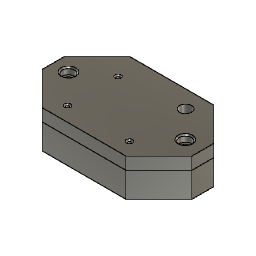
feet mold (Autodesk Fusion 360 design; units mm, degrees)
Autodesk Fusion 360 part; units mm, degrees
note: some values were not read from the file. Chosen so that the rebuilt part matches the saved one: which bodies a step acts on; which face or edge a step refers to. Set by a fixed rule: which sketch regions a step uses.
sketch "base" plane through (0, 0, 0) normal (0, 0, 1) x (1, 0, 0)
  circle A0 centre (0, 0) radius 2.65
  circle A1 centre (0, 0) radius 5
  line L0 (-10, 18.1) -> (18.1, 18.1)
  line L1 (18.1, 18.1) -> (18.1, -10)
  line L2 (18.1, -10) -> (-10, -10)
  line L3 (-10, -10) -> (-10, 18.1)
  line L4 (0, 0) -> (0, 20) construction
  arc A2 (-4.8405, 18.1) -> (4.8405, 18.1) centre (0, 20) ccw
  line L5 (-10, 15.5) -> (-7.4, 18.1)
  line L6 (-10, -7.4) -> (-7.4, -10)
  line L7 (18.1, -7.4) -> (15.5, -10)
  line L8 (-10, -7.4) -> (18.1, -7.4) construction
  line L9 (-7.4, 18.1) -> (-7.4, -10) construction
  arc A3 (18.1, 4.8405) -> (18.1, -4.8405) centre (20, 0) ccw
  line L10 (0, 0) -> (20, 0) construction
  line L11 (-2.2249, 15.3) -> (2.2249, 15.3)
  line L12 (15.3, 2.2249) -> (15.3, -2.2249)
  line L13 (-30, 26) -> (38.1, 26)
  line L14 (38.1, 26) -> (38.1, -14)
  line L15 (38.1, -14) -> (-30, -14)
  line L16 (-30, -14) -> (-30, 26)
  circle A4 centre (-23, 6) radius 2.75
  circle A5 centre (-23, 6) radius 1.6
  line L17 (-19.7, 6) -> (-21.35, 8.8579)
  line L18 (-21.35, 8.8579) -> (-24.65, 8.8579)
  line L19 (-24.65, 8.8579) -> (-26.3, 6)
  line L20 (-26.3, 6) -> (-24.65, 3.1421)
  line L21 (-24.65, 3.1421) -> (-21.35, 3.1421)
  line L22 (-21.35, 3.1421) -> (-19.7, 6)
  circle A6 centre (30.1, 6) radius 1.6
  circle A7 centre (30.1, 6) radius 2.75
  line L23 (33.4, 6) -> (31.75, 8.8579)
  line L24 (31.75, 8.8579) -> (28.45, 8.8579)
  line L25 (28.45, 8.8579) -> (26.8, 6)
  line L26 (26.8, 6) -> (28.45, 3.1421)
  line L27 (28.45, 3.1421) -> (31.75, 3.1421)
  line L28 (31.75, 3.1421) -> (33.4, 6)
  circle A8 centre (-10, 15.5) radius 0.75
  circle A9 centre (-10, -7.4) radius 0.75
  circle A10 centre (18.1, 18.1) radius 2.325
  circle A11 centre (18.1, -7.4) radius 0.75
  point P0 (-23, 6)
  point P1 (30.1, 6)
  dimension "d5" = 5.3
  dimension "d6" = 10
  dimension "d7" = 10
  dimension "d12" = 10
  dimension "d13" = 5.2
  dimension "d14" = 2.6
  dimension "d27" = 20
  dimension "d59" = 45
  dimension "d61" = 45
  dimension "d62" = 45
  dimension "d68" = 5.2
  dimension "d69" = 20
  dimension "d70" = 28.1
  dimension "d81" = 1.9
  dimension "d88" = 0.5
  dimension "d89" = 0.5
  dimension "d94" = 25.5
  dimension "d95" = 68.1
  dimension "d96" = 40
  dimension "d97" = 20
  dimension "d107" = 5.5
  dimension "d108" = 3.2
  dimension "d109" = 3.3
  dimension "d110" = 3.2
  dimension "d111" = 5.5
  dimension "d112" = 3.3
  dimension "d113" = 20
  dimension "d114" = 20
  dimension "d115" = 7
  dimension "d116" = 8
  dimension "d127" = 1.5
  dimension "d128" = 1.5
  dimension "d130" = 4.65
  dimension "d139" = 1.5
  constraint coincident A0.centre A1.centre
  constraint concentric A0 A1
  constraint horizontal L0
  constraint vertical L1
  constraint horizontal L2
  constraint vertical L3
  constraint perpendicular L0 L4
  constraint coincident L0 A2.end
  constraint coincident L0 A2.start
  constraint coincident L4.end A2.centre
  constraint coincident L3 L5.start
  constraint coincident L0 L5.end
  constraint coincident L2 L6.end
  constraint coincident L3 L6.start
  constraint coincident L2 L7.end
  constraint coincident L1 L7.start
  constraint perpendicular L3 L8
  constraint perpendicular L2 L9
  constraint coincident L1 A3.end
  constraint coincident L1 A3.start
  constraint coincident A3.centre L10.end
  constraint perpendicular L4 L10
  constraint equal L2 L3
  constraint coincident A2 L11.end
  constraint perpendicular L4 L11
  constraint coincident A2 L11.start
  constraint coincident A3 L12.start
  constraint coincident A3 L12.end
  constraint perpendicular L10 L12
  constraint horizontal L13
  constraint vertical L14
  constraint horizontal L15
  constraint vertical L16
  constraint concentric A4 A5
  constraint coincident P0 A4.centre
  constraint concentric A6 A7
  constraint coincident P1 A6.centre
  constraint coincident L5.start A8.centre
  constraint coincident L6.start L8.start
  constraint coincident L0.end L1.start
  constraint coincident L7.start L8.end
  measures "d5" diameter of A0
  measures "d6" diameter of A1
  measures "d7" vertical distance of A0.centre L1.end
  measures "d12" horizontal distance of L0.start L4.end
  measures "d13" radius of A2
  measures "d14" horizontal distance of L0.start L5.end
  measures "d27" vertical distance of A0.centre L4.end
  measures "d59" angle of L2 L7
  measures "d61" angle of L0 L5
  measures "d62" angle of L2 L6
  measures "d68" radius of A3
  measures "d69" distance of A0.centre A3.centre
  measures "d70" distance of L0.start L2.end
  measures "d81" distance of L0 L4.end
  measures "d88" distance of A2 L11
  measures "d89" distance of A3 L12
  measures "d94" distance of L0.start L6.start
  measures "d95" distance of L13.start L13.end
  measures "d96" distance of L13.start L15.end
  measures "d97" distance of L3 L16
  measures "d107" diameter of A4
  measures "d108" diameter of A5
  measures "d109" distance of L17.start P0
  measures "d110" diameter of A6
  measures "d111" diameter of A7
  measures "d112" distance of L23.start P1
  measures "d113" distance of L15 P1
  measures "d114" distance of L15 P0
  measures "d115" distance of L16 P0
  measures "d116" distance of L14 P1
  measures "d127" diameter of A8
  measures "d128" diameter of A9
  measures "d130" diameter of A10
  measures "d139" diameter of A11
extrude "Extrude1" add sketch "base" along normal blind 6.4 contours L0 L1 L2 L3 A2 L5 L6 L7 A3 A8 A9 A10 A11 | L3 L5 A8 | A2 L11 | L3 L6 A9 | L0 L1 A10 | A3 L12 | L1 L7 A11 picked at (-9.6473, 15.1473) picked at (-9.6007, -7.1011) picked at (16.5579, 17.9897) picked at (18.0633, -6.9027) makes body 1
extrude "Extrude2" add sketch "base" along normal blind 3 contours A1 bodies 1
extrude "Extrude3" add sketch "base" along normal blind 2.6 contours L0 L3 L5 A8 | L0 L1 L2 L3 A2 L5 L6 L7 A3 A8 A9 A10 A11 | L3 L5 A8 | L0 A2 L11 | L3 L5 A8 | A2 L11 | L3 L6 A9 | L0 L1 A10 | L3 L6 A9 | L2 L3 L6 A9 | L1 A3 L12 | A3 L12 | L1 L2 L7 A11 | L1 L7 A11 | L1 L7 A11 picked at (16.5579, 17.9897) bodies 1
extrude "Extrude11" cut sketch "base" along normal up to surface (5.4 mm away) contours L0 A2 L11 | A2 L11 | L1 A3 L12 | A3 L12 bodies 1
draft "Draft2" angle 45 neutral plane through (-10, -7.4, 0) pull (-0.707107, -0.707107, 0) 1 faces at (-9.1333, -9.1333, 2.6) on bodies 1
draft "Draft3" angle 45 neutral plane through (18.1, -7.4, 0) pull (0.707107, -0.707107, 0) 1 faces at (17.2333, -9.1333, 2.6) on bodies 1
draft "Draft5" angle 45 neutral plane through (-10, 15.5, 0) pull (-0.707107, 0.707107, 0) 1 faces at (-9.1333, 17.2333, 2.6) on bodies 1
draft "Draft8" angle 45 neutral plane through (15.3, 2.2249, 0) pull (1, 0, 0) 1 faces at (15.2081, 0.5035, 5.4) on bodies 1
draft "Draft9" angle 45 neutral plane through (-2.2249, 15.3, 0) pull (0, 1, 0) 1 faces at (0.5035, 15.2081, 5.4) on bodies 1
sketch "selective_infill" plane through (0, 0, 0) normal (0, 0, -1) x (1, 0, 0)
  line L0 (-10, -18.1) -> (-4.8405, -18.1)
  line L1 (18.1, 4.8405) -> (18.1, 10)
  line L2 (18.1, 10) -> (-10, 10)
  line L3 (-10, 10) -> (-10, -18.1)
  circle A0 centre (0, 0) radius 2.65
  line L4 (4.7284, 2.65) -> (4.8294, 2.65)
  line L5 (4.8294, 2.65) -> (4.8294, -2.65)
  line L6 (4.8294, -2.65) -> (4.7284, -2.65)
  line L7 (4.7284, -2.65) -> (4.7284, 2.65)
  line L8 (-4.7284, 2.65) -> (-4.8294, 2.65)
  line L9 (-4.8294, 2.65) -> (-4.8294, -2.65)
  line L10 (-4.8294, -2.65) -> (-4.7284, -2.65)
  line L11 (-4.7284, -2.65) -> (-4.7284, 2.65)
  line L12 (-4.7284, 0) -> (4.7284, 0) construction
  arc A1 (18.1, 4.8405) -> (18.1, -4.8405) centre (20, 0) ccw
  arc A2 (4.8405, -18.1) -> (-4.8405, -18.1) centre (0, -20) ccw
  circle A3 centre (0, 0) radius 2.65
  line L13 (4.8405, -18.1) -> (18.1, -18.1)
  line L14 (18.1, -18.1) -> (18.1, -4.8405)
  dimension "d52" = 0.101
  dimension "d53" = 0.101
  constraint horizontal L4
  constraint vertical L5
  constraint horizontal L6
  constraint vertical L7
  constraint horizontal L8
  constraint vertical L9
  constraint horizontal L10
  constraint vertical L11
  constraint midpoint L11 L12.start
  constraint midpoint L7 L12.end
  constraint perpendicular L7 L12
  constraint coincident A0.centre L12
  constraint tangent A0 L10
  constraint tangent A0 L6
  measures "d52" distance of L8.start L8.end
  measures "d53" horizontal distance of L4.start L4.end
extrude "Extrude9" cut sketch "selective_infill" along normal up to surface (0.8 mm away) from surface at -1.8 contours L4 L5 L6 L7 | L8 L9 L10 L11 bodies 1
extrude "Extrude12" add sketch "base" against normal blind 5 separate body contours A0 | A1 | L0 L3 L5 A8 | L0 L1 L2 L3 A2 L5 L6 L7 A3 A8 A9 A10 A11 | L3 L5 A8 | L3 A8 | L0 A2 L11 | L3 L5 A8 | A2 L11 | L3 L6 A9 | L3 A9 | L0 L1 A10 | L0 L1 A10 | L3 L6 A9 | L2 L3 L6 A9 | L1 A3 L12 | A3 L12 | L1 L2 L7 A11 | L1 A11 | L1 L7 A11 | L1 L7 A11 | L13 L14 L15 L16 | A4 | A5 | L17 L18 L19 L20 L21 L22 | A6 | A7 | L23 L24 L25 L26 L27 L28 makes body 2
extrude "Extrude13" add 1 faces at (-7.3, -0.6667, 0) along direction (0, 0, 1) blind 12 separate body on bodies 2 makes body 3
combine "Combine1" operation add target body 2 tool bodies 3
combine "Combine2" operation cut target body 2 tool bodies 1 makes body 4 at (-4.8294, -0.8833, 1.5333) makes body 5 at (4.7284, 0.8833, 1.5333)
ref_plane "WorkPlane5" through (4.05, 6, 6.4) normal (0, 0, 1) x (1, 0, 0)
split "Split1" by plane through (4.05, 6, 6.4) normal (0, 0, 1) bodies 2 makes body 6 at (-7.3, -0.6667, 12)
extrude "Extrude14" add 1 faces at (-1.3771, -0.9389, 6.4) along direction (0, 0, -1) up to surface (3.4 mm away) separate body on bodies 2 makes body 7
combine "Combine3" operation add target body 6 tool bodies 7
extrude "Extrude15" cut 1 faces at (-1.3771, -0.9389, 6.4) along direction (0, 0, -1) up to surface (3.4 mm away) on bodies 2 bodies 2
extrude "Extrude16" cut sketch "base" along normal blind 50 and the other way blind 50 contours A5 | A6 bodies 2 6
extrude "Extrude17" cut sketch "base" against normal blind 3 from surface at 12 contours A4 | A7 bodies 6
extrude "Extrude18" cut sketch "base" along normal blind 2.8 from surface at -5 contours A4 | L17 L18 L19 L20 L21 L22 | A7 | L23 L24 L25 L26 L27 L28 bodies 2
extrude "Extrude19" cut sketch "base" along normal blind 40 from surface at 6.4 contours L3 L5 A8 | L3 A8 | L3 L5 A8 | L3 L6 A9 | L3 A9 | L0 L1 A10 | L0 L1 A10 | L3 L6 A9 | L1 A11 | L1 L7 A11 | L1 L7 A11 bodies 6
chamfer "Chamfer2" distance 0.4 distance2 4 1 edges at (15.9323, 18.9408, 12) measured on face at (8.1652, 8.2062, 12) on bodies 6
chamfer "Chamfer3" distance 15 angle 45 8 edges at (-30, 26, 9.2) (38.1, 26, 9.2) (-30, -14, 9.2) (38.1, -14, 9.2) (-30, 26, 0.7) (38.1, 26, 0.7) (-30, -14, 0.7) (38.1, -14, 0.7) on bodies 2 6
chamfer "Chamfer4" distance 0.6 angle 45 5 edges at (-10.6992, 15.7712, 12) (-10.6992, -7.1288, 12) (17.4008, -7.1288, 12) (27.5361, 6.9944, 12) (-25.5639, 6.9944, 12) on bodies 6
hidden bodies 4 5
equation "m5_hole = 5.3 mm"
equation "m5_head = 10 mm"
equation "foot_thickness = 6.4 mm"
equation "corner_angle = 45 °"
equation "d5 = m5_hole"
equation "d6 = m5_head"
equation "d13 = m5_head / 2 + 0.2 mm"
equation "d18 = foot_thickness"
equation "layer_height = 0.20 mm"
equation "e_width = 0.45 mm"
equation "num_perimeters = 3"
equation "num_top_bottom = 5"
equation "perimeters_thickness = e_width + ( num_perimeters * 2 - 1 ) * 0.4071 mm"
equation "top_bottom_thickness = num_top_bottom * layer_height"
equation "d54 = -top_bottom_thickness - layer_height * 4"
equation "d57 = -top_bottom_thickness"
equation "d59 = 45 °"
equation "d61 = 45 °"
equation "d62 = 45.00 °"
equation "e_spacing = 0.4071 mm"
equation "d68 = m5_head / 2 + 0.2 mm"
equation "d72 = 45 °"
equation "d73 = 0.0 °"
equation "d74 = 45.0 °"
equation "d75 = 0.0 °"
equation "d78 = 45.0 °"
equation "d79 = 0.0 °"
equation "d90 = 45.0 °"
equation "d91 = 0.0 °"
equation "d92 = 45.0 °"
equation "d93 = 0.0 °"
equation "d120 = 0.0 °"
equation "d127 = ventHoles"
equation "d128 = ventHoles"
equation "ventHoles = 1.5 mm"
equation "d139 = ventHoles"
